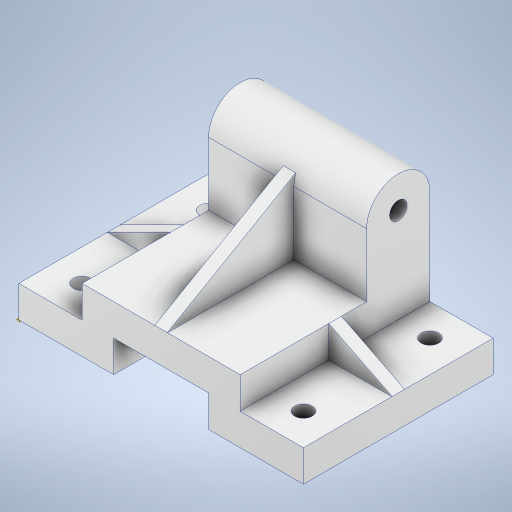
# Autodesk Inventor part: Homework 1d
Saved by Autodesk Inventor 2024 (Build 280153000, 153)
## iProperties
Created: 2023-08-26
Part Number: Homework 1d
Material: Aluminum 6061
Document SubType Name: Modeling
Designer: Nate
Density: 2.7 g/cm^3
Appearance: Aluminum - Flat
Mass: 254.787 g
Surface Area: 227.998 cm^2
Volume: 94.3657 cm^3
Author: Nate
Autodesk Inventor part; units mm, degrees
ref_plane "XZ Plane" through (0, 0, 0) normal (0, 1, 0) x (-1, 0, 0)
sketch "Sketch1" plane through (0, 0, 0) normal (0, 1, 0) x (-1, 0, 0)
  line L0 (0, 0) -> (-90, 0)
  line L1 (-90, 0) -> (-90, -60)
  line L2 (-90, -60) -> (0, -60)
  line L3 (0, -60) -> (0, 0)
  line L4 (-30, 0) -> (-60, 0)
  line L5 (-60, 0) -> (-60, -60)
  line L6 (-60, -60) -> (-30, -60)
  line L7 (-30, -60) -> (-30, 0)
  line L8 (-20, -60) -> (-70, -60)
  line L9 (-70, -60) -> (-70, 0)
  line L10 (-70, 0) -> (-20, 0)
  line L11 (-20, 0) -> (-20, -60)
  line L12 (-20, -60) -> (-70, -60)
  line L13 (-70, -60) -> (-70, -40)
  line L14 (-70, -40) -> (-20, -40)
  line L15 (-20, -40) -> (-20, -60)
  circle A0 centre (-10, -50) radius 2.75
  circle A1 centre (-10, -10) radius 2.75
  circle A2 centre (-80, -50) radius 2.75
  circle A3 centre (-80, -10) radius 2.75
  point P0 (0, -30)
  point P1 (-60, -40)
  point P2 (-30, -40)
  point P3 (-70, 0)
  point P4 (-20, 0)
  dimension "d0" = 90
  dimension "d1" = 60
  dimension "d2" = 30
  dimension "d3" = 30
  dimension "d4" = 50
  dimension "d5" = 60
  dimension "d6" = 20
  dimension "d7" = 20
  dimension "d8" = 5.5
  dimension "d9" = 5.5
  dimension "d10" = 5.5
  dimension "d11" = 5.5
  dimension "d12" = 10
  dimension "d13" = 10
  dimension "d14" = 10
  dimension "d15" = 10
  dimension "d16" = 10
  dimension "d17" = 10
  dimension "d18" = 10
  dimension "d19" = 10
  constraints: 32 end point, 8 parallel, 4 centre point, 4 horizontal, 4 perpendicular, 4 point on line, 1 midpoint
  measures "d0" distance of L2.end L1.end
  measures "d1" distance of L1.end L0.end
  measures "d2" distance of L6.end L5.end
  measures "d3" distance from line of L7 point (0, -30)
  measures "d4" distance of L9.end L10.end
  measures "d5" distance of L8.end L9.end
  measures "d6" distance between parallel lines of L11 L3
  measures "d7" distance between parallel lines of L12 L14
  measures "d8" diameter of A0
  measures "d9" diameter of A1
  measures "d10" diameter of A2
  measures "d11" diameter of A3
  measures "d12" distance from line of A0.centre L2
  measures "d13" distance from line of A0.centre L3
  measures "d14" distance from line of A1.centre L3
  measures "d15" distance from line of A1.centre L0
  measures "d16" distance from line of L2 A2.centre
  measures "d17" distance from line of L1 A2.centre
  measures "d18" distance from line of L1 A3.centre
  measures "d19" distance from line of A3.centre L0
extrude "Extrusion1" add sketch "Sketch1" along normal blind 10 contours L3 L2 L11 L0 | L9 L2 L1 L0
extrude "Extrusion2" add sketch "Sketch1" along normal blind 20 contours L11 L14 L7 L0 | L7 L14 L5 L0 | L11 L2 L7 L14 | L5 L14 L9 L0 | L5 L2 L9 L14
extrude "Extrusion3" add sketch "Sketch1" along normal blind 50 contours L11 L2 L7 L14 | L7 L2 L5 L14 | L5 L2 L9 L14
extrude "Extrusion4" cut sketch "Sketch1" along normal blind 10 contours L7 L14 L5 L0 | L7 L2 L5 L14
ref_plane "Work Plane2" through (0, 0, -30) normal (0, 0, 1) x (1, 0, 0)
ref_plane "Work Plane3" through (45, 0, 0) normal (1, 0, 0) x (0, 1, 0)
sketch "Sketch7" plane through (0, 0, -30) normal (0, 0, 1) x (1, 0, 0)
  line L0 (20, 10) -> (20, 20) projected
  line L1 (20, 10) -> (0, 10) projected
  line L2 (20, 20) -> (0, 10)
  line L3 (0, 10) -> (20, 10)
  line L4 (20, 10) -> (20, 20)
  line L5 (70, 20) -> (60, 20) projected
  line L6 (70, 20) -> (90, 10)
  line L7 (90, 10) -> (70, 10) projected
  line L8 (90, 10) -> (70, 10)
  line L9 (70, 10) -> (70, 20)
  point P0 (0, 0)
  constraints: 12 end point, 2 collinear, 2 perpendicular
extrude "Extrusion9" add sketch "Sketch7" along normal mid plane 4
sketch "Sketch8" plane through (45, 0, 0) normal (1, 0, 0) x (0, 1, 0)
  circle A0 centre (40, -50) radius 2.75
  line L0 (20, 0) -> (50, -51.9582)
  line L1 (20, 0) -> (20, -51.9582)
  line L2 (20, -51.9582) -> (50, -51.9582)
  point P0 (0, 0)
  point P1 (38.0692, -51.9582)
  point P2 (41.9308, -51.9582)
  dimension "d45" = 40
  dimension "d49" = 50
  dimension "d50" = 20
  dimension "d55" = 5.5
  constraints: 6 end point, 1 centre point, 1 perpendicular, 1 vertical
  measures "d45" horizontal distance of A0.centre point (0, 0)
  measures "d49" horizontal distance of point (0, 0) L0.end
  measures "d50" distance of L0.start point (0, 0)
  measures "d55" diameter of A0
extrude "Extrusion10" add sketch "Sketch8" along normal mid plane 4 contours A0 L2 L1 L0
extrude "Extrusion11" cut sketch "Sketch8" along normal through all both and the other way through all contours A0 L2 | L2 A0
fillet "Fillet1" radius 10 2 edges at (45, 50, -40) (45, 50, -60)
body "Solid1"
